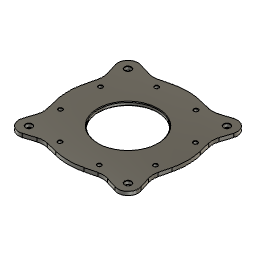
Fitment v1 (Autodesk Fusion 360 archive; units mm, degrees)
design "Motor_Base_Plate_Top v4"
Autodesk Fusion 360 part; units mm, degrees
sketch "Sketch1" plane through (0, 0, 0) normal (0, 0, 1) x (1, 0, 0)
  line L0 (49, 49) -> (-49, 49) construction
  line L1 (-49, 49) -> (-49, -49) construction
  line L2 (-49, -49) -> (49, -49) construction
  line L3 (49, -49) -> (49, 49) construction
  line L4 (49, 49) -> (-49, -49) construction
  line L5 (-49, 49) -> (49, -49) construction
  line L6 (-34.6482, 34.6482) -> (-33.8425, 35.454)
  line L7 (-34.6482, 34.6482) -> (-20.2965, 49) construction
  line L8 (-34.6482, 34.6482) -> (-49, 20.2965) construction
  line L9 (-34.6482, -34.6482) -> (-49, -20.2965) construction
  line L10 (-34.6482, -34.6482) -> (-20.2965, -49) construction
  line L11 (34.6482, -34.6482) -> (20.2965, -49) construction
  line L12 (34.6482, -34.6482) -> (49, -20.2965) construction
  line L13 (34.6482, 34.6482) -> (49, 20.2965) construction
  line L14 (34.6482, 34.6482) -> (20.2965, 49) construction
  line L15 (-20.8111, 45.3788) -> (-11.5222, 47.626)
  line L16 (-28.9236, 45.6762) -> (-38.023, 48.5976)
  arc A0 (-28.9236, 45.6762) -> (-20.8111, 45.3788) centre (-24.3383, 59.9582) ccw
  arc A1 (-45.3788, 20.8111) -> (-45.6762, 28.9236) centre (-59.9582, 24.3383) ccw
  line L17 (-45.6762, 28.9236) -> (-48.5976, 38.023)
  line L18 (-45.3788, 20.8111) -> (-47.626, 11.5222)
  line L19 (-45.6762, -28.9236) -> (-48.5976, -38.023)
  line L20 (-28.9236, -45.6762) -> (-38.023, -48.5976)
  arc A2 (-20.8111, -45.3788) -> (-28.9236, -45.6762) centre (-24.3383, -59.9582) ccw
  line L21 (-20.8111, -45.3788) -> (-11.5222, -47.626)
  arc A3 (-45.6762, -28.9236) -> (-45.3788, -20.8111) centre (-59.9582, -24.3383) ccw
  line L22 (-45.3788, -20.8111) -> (-47.626, -11.5222)
  line L23 (28.9236, -45.6762) -> (38.023, -48.5976)
  line L24 (45.6762, -28.9236) -> (48.5976, -38.023)
  arc A4 (45.3788, -20.8111) -> (45.6762, -28.9236) centre (59.9582, -24.3383) ccw
  line L25 (45.3788, -20.8111) -> (47.626, -11.5222)
  arc A5 (28.9236, -45.6762) -> (20.8111, -45.3788) centre (24.3383, -59.9582) ccw
  line L26 (20.8111, -45.3788) -> (11.5222, -47.626)
  line L27 (45.6762, 28.9236) -> (48.5976, 38.023)
  line L28 (28.9236, 45.6762) -> (38.023, 48.5976)
  arc A6 (20.8111, 45.3788) -> (28.9236, 45.6762) centre (24.3383, 59.9582) ccw
  line L29 (20.8111, 45.3788) -> (11.5222, 47.626)
  arc A7 (45.6762, 28.9236) -> (45.3788, 20.8111) centre (59.9582, 24.3383) ccw
  line L30 (45.3788, 20.8111) -> (47.626, 11.5222)
  arc A8 (-38.023, 48.5976) -> (-48.5976, 38.023) centre (-40.5929, 40.5929) ccw
  arc A9 (-48.5976, -38.023) -> (-38.023, -48.5976) centre (-40.5929, -40.5929) ccw
  arc A10 (38.023, -48.5976) -> (48.5976, -38.023) centre (40.5929, -40.5929) ccw
  arc A11 (48.5976, 38.023) -> (38.023, 48.5976) centre (40.5929, 40.5929) ccw
  arc A12 (11.5222, 47.626) -> (-11.5222, 47.626) centre (0, 0) ccw
  arc A13 (47.626, -11.5222) -> (47.626, 11.5222) centre (0, 0) ccw
  arc A14 (-47.626, 11.5222) -> (-47.626, -11.5222) centre (0, 0) ccw
  arc A15 (-11.5222, -47.626) -> (11.5222, -47.626) centre (0, 0) ccw
  circle A16 centre (-40.5929, 40.5929) radius 2.5
  circle A17 centre (-40.5929, -40.5929) radius 2.5
  circle A18 centre (40.5929, -40.5929) radius 2.5
  circle A19 centre (40.5929, 40.5929) radius 2.5
  circle A20 centre (0, 0) radius 42.5 construction
  line L31 (0, 0) -> (16.6061, 39.1215) construction
  line L32 (0, 0) -> (42.5, 0) construction
  circle A21 centre (16.6061, 39.1215) radius 1.5
  circle A22 centre (-15.9208, 39.4053) radius 1.5
  circle A23 centre (-39.1215, 16.6061) radius 1.5
  circle A24 centre (-39.4053, -15.9208) radius 1.5
  circle A25 centre (-16.6061, -39.1215) radius 1.5
  circle A26 centre (15.9208, -39.4053) radius 1.5
  circle A27 centre (39.1215, -16.6061) radius 1.5
  circle A28 centre (39.4053, 15.9208) radius 1.5
  circle A29 centre (0, 0) radius 24.25
  dimension "d1" = 98
  dimension "d2" = 98
  dimension "d3" = 98
  dimension "d5" = 360
  dimension "d8" = 15
  dimension "d12" = 360
  dimension "d13" = 5
  dimension "d15" = 360
  dimension "d18" = 85
  dimension "d19" = 67
  dimension "d20" = 3
  dimension "d22" = 360
  dimension "d23" = 48.5
  constraint coincident A12.centre A13.centre
  constraint horizontal L0
  constraint perpendicular L0 L1
  constraint parallel L0 L2
  constraint parallel L1 L3
  constraint coincident L4 A12.centre
  constraint coincident L5 A12.centre
  constraint coincident L5 L6.start
  constraint tangent L6 A14
  constraint tangent L7 A14
  constraint symmetric L5 L6.start L7.start
  constraint symmetric L5 L7.end L8.end
  constraint tangent L15 A14
  constraint tangent L16 A0
  constraint tangent L15 A0
  constraint symmetric L5 L15.end L18.end
  constraint symmetric L5 L16.end L17.end
  constraint symmetric L5 L16.start A1.end
  constraint symmetric L5 L15.start A1.start
  constraint symmetric L5 A0 A1
  constraint tangent L0 A8
  constraint tangent L1 A8
  constraint tangent L8 A8
  constraint concentric A12 A14
  constraint concentric A13 A14
  constraint concentric A14 A15
  constraint concentric A8 A16
  constraint concentric A14 A20
  constraint horizontal L32
  constraint coincident A20 L31.end
  constraint coincident L31.end A21.centre
  constraint concentric A12 A29
  measures "d1" diameter of A14
  measures "d2" distance of L1.end L2.end
  measures "d3" distance of L0.end L1.end
  measures "d8" radius of A0
  measures "d13" diameter of A16
  measures "d18" diameter of A20
  measures "d19" angle of L31 L32
  measures "d20" diameter of A21
  measures "d23" diameter of A29
extrude "Extrude1" add sketch "Sketch1" along normal blind 3
chamfer "Chamfer1" distance 0.5 angle 45 1 faces at (-24.2199, -1.2088, 2)
chamfer "Chamfer1" distance 0.25 angle 45 12 faces at (-38.096, 40.4683, 2) (-38.7152, 15.1621, 1) (-37.9072, -15.9955, 2) (-17.2381, 38.6879, 2) (17.886, 39.9036, 2) (39.8116, 14.4768, 1) (43.0898, 40.4683, 2) (43.0898, -40.7175, 2) (38.4371, -17.9409, 2) (17.2007, -38.6232, 2) (-17.9234, -39.8388, 2) (-38.096, -40.7175, 2)
equation "d3 = 120 mm - 2 mm - 20 mm"
equation "d19 = 90 deg - 23 deg"
